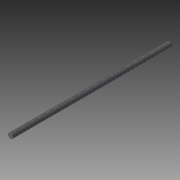
# Autodesk Inventor part: threaded_rod
Saved by Autodesk Inventor 2014 SP2 (Build 180246200, 246)
## iProperties
Created: 2014-07-14
Part Number: threaded_rod
Material: Generic
Document SubType Name: Modeling
Designer: cruiser
Density: 1 g/cm^3
Appearance: Default
Mass: 12.5664 g
Surface Area: 63.8372 cm^2
Volume: 12.5664 cm^3
Author: cruiser
Autodesk Inventor part; units mm, degrees
ref_plane "YZ Plane" through (0, 0, 0) normal (1, 0, 0) x (0, 1, 0)
ref_plane "XZ Plane" through (0, 0, 0) normal (0, 1, 0) x (-1, 0, 0)
ref_plane "XY Plane" through (0, 0, 0) normal (0, 0, 1) x (1, 0, 0)
sketch "Sketch1" plane through (0, 0, 0) normal (0, 1, 0) x (-1, 0, 0)
  circle A0 centre (0, 0) radius 4
  dimension "d0" = 8
  constraints: 1 centre point, 1 coincident
  measures "d0" diameter of A0
extrude "Extrusion1" add sketch "Sketch1" along normal blind 250
thread "Thread1" size "M8x1.25" class "6g" standard "ISO Metric profile" full length
equation "\"sm_thickness\" = 1.5875"
equation "\"very_thick_acrylic\" = 9.45"
equation "\"thick_acrylic\" = 5.88"
equation "\"thin_acrylic\" = 3.15"
equation "\"clear_acrylic\" = 3.15"
equation "\"wood_thickness\" = 6.72"
equation "\"m3_diameter\" = 3"
equation "\"m3_head\" = 6"
equation "\"m4_diameter\" = 4"
equation "\"m5_diameter\" = 5"
equation "\"m5_head\" = 10.3"
equation "\"brass_insert_drill\" = 4"
equation "\"m5_brass_insert_drill\" = 6.7"
equation "\"m3_press_nut_drill\" = 4.5"
equation "\"m5_press_nut_drill\" = 6.5"
equation "\"m3_main_length\" = 14"
equation "\"m3_main_nut_width\" = 5.7"
equation "\"m3_main_nut_thickness\" = 2.5"
equation "\"m3_main_extra\" = 1"
equation "\"stepper_screw_space\" = 35"
equation "\"stepper_shaft_diameter\" = 5"
equation "\"stepper_body_diameter\" = 28"
equation "\"laser_body_diameter\" = 12"
equation "\"carrier_y\" = 251"
equation "\"carrier_z\" = 12"
equation "\"visor_x\" = 253.925"
equation "\"visor_y\" = 85.6"
equation "\"window_z\" = 332.225"
equation "\"window_y\" = 93.75"
equation "\"window_overlap\" = 48"
equation "\"acrylic_into_frame\" = 5"
equation "\"door_x\" = 251"
equation "\"door_z\" = 332.225"
equation "\"door_overlap\" = 48"
equation "\"reservoir_z\" = 35"
equation "\"linear_bearing_spacing\" = 209"
equation "\"motor_spacing\" = 337"
equation "\"tray_border\" = 25"
equation "\"bed_z\" = 25"
equation "\"crane_x\" = 234"
equation "\"crane_z2\" = 12"
equation "\"end_stop_spacing\" = 19"
equation "\"thumb_nut_offset_y\" = 0"
equation "\"thumb_nut_diameter\" = 7"
equation "\"z_min_from_center\" = 115"
equation "\"frame_top_z\" = 385"
equation "\"frame_bottom_z\" = 275"
equation "\"frame_total_z\" = 661.5875"
equation "\"frame_foot_z\" = 12"
equation "\"frame_tilt\" = 1deg"
equation "\"printer_z\" = 289"
equation "\"lcd_x\" = 72"
equation "\"lcd_y\" = 25"
equation "\"subframe_x\" = 66"
equation "\"subframe_y_offset\" = 27.5"
equation "\"laser_y_offset\" = 19.4"
equation "\"laser_diameter\" = 13"
equation "\"laser_z_offset\" = 55"
equation "\"laser_y\" = 15"
equation "\"laser_z\" = 75"
equation "\"t_galvo_frame\" = 6.72"
equation "\"galvo_frame_x\" = 66"
equation "\"galvo_frame_z\" = 85"
equation "\"galvo_frame_y_offset\" = 27.5"
equation "\"drawer_x\" = 202.02372"
equation "\"drawer_y\" = 72"
equation "\"drawer_z_from_bottom\" = 25"
equation "\"nema17_x\" = 43"
equation "\"drawer_support_from_top\" = 48"
equation "\"laser_gap\" = 1"
equation "\"frame_screw_from_center\" = 25"
equation "\"drawer_screw_from_center\" = 55"
equation "\"frame_face_y\" = 45"
equation "\"switch_spacing\" = 19"
equation "\"subframe_y\" = 55"
equation "\"al_thickness\" = 1.5875"
equation "\"rivet_diameter\" = 3.3"
equation "\"bend_factor\" = 2.26205"
equation "\"sm_bend\" = 3.591"
equation "\"al_bend\" = 3.591"
equation "\"frame_x\" = 353.375"
equation "\"carrier_z2\" = 25"
equation "\"carrier_y2\" = 76.825"
equation "\"injection_plastic\" = 3.15"
equation "\"subframe_t\" = 0.79375"
equation "\"laser_offset_y\" = 8.5"
equation "\"laser_offset_x\" = 59.5"
equation "\"laser_holder_z\" = 75"
equation "\"laser_holder_t\" = 0.79375"
equation "\"foot_x\" = 192"
equation "\"foot_y\" = 194"
equation "\"foot_t\" = 1.5875"
equation "\"lmk8uu_x\" = 25"
equation "\"galvo_y_out_offset\" = 27"
equation "\"lmk8uu_z\" = 24"
equation "\"acme_nut_upper_d\" = 12.7"
equation "\"frame_front_x\" = 280.23622"
equation "\"frame_front_fold\" = 15"
equation "\"reservoir_t\" = 0.79375"
equation "\"platform_z\" = 65"
equation "\"platform_fold_x\" = 15"
equation "\"platform_upper_y\" = 46.625"
equation "\"tray_to_platform_oversize\" = 0"
equation "\"frame_back_t\" = 0.91186"
equation "\"frame_gap\" = 0.1"
equation "\"drawer_reservoir_overlap_x\" = 24.20625"
equation "\"frame_front_t\" = 0.91186"
equation "\"frame_back_z\" = 497.97628"
equation "\"frame_back_y\" = 53.97628"
equation "\"frame_back_x\" = 278.2125"
equation "\"drawer_gap\" = 0.1"
equation "\"drawer_t\" = 0.79375"
equation "\"frame_opening_x\" = 200.23622"
equation "\"drawer_window_gap\" = 5"
equation "\"acme_nut_d\" = 19.1"
equation "\"shf8_y\" = 43"
equation "\"galvo_y_in_offset\" = 17.5"
equation "\"nema17_shaft\" = 24"
equation "\"lmk8uu_shaft\" = 15"
equation "\"reservoir_flap_y\" = 20.79375"
body "Solid1"
